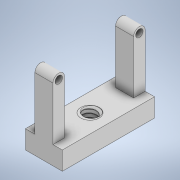
# Autodesk Inventor part: hires mount for beamsplitter test
Saved by Autodesk Inventor 2022 (Build 260153000, 153)
## iProperties
Created: 2022-07-06
Part Number: hires mount for beamsplitter test
Material: Generic
Document SubType Name: Modeling
Designer: Eli
Density: 1 g/cm^3
Appearance: Default
Author: Eli
Autodesk Inventor part; units mm, degrees
note: some values were not read from the file. Chosen so that the rebuilt part matches the saved one: direction of "Hole1"; direction of "Hole2".
ref_plane "YZ Plane" through (0, 0, 0) normal (1, 0, 0) x (0, 1, 0)
ref_plane "XZ Plane" through (0, 0, 0) normal (0, 1, 0) x (-1, 0, 0)
sketch "Sketch1" plane through (0, 0, 0) normal (0, 1, 0) x (-1, 0, 0)
  line L0 (0, 0) -> (-12.7, 0)
  line L1 (-12.7, 0) -> (-12.7, -31.75)
  line L2 (-12.7, -31.75) -> (0, -31.75)
  line L3 (0, -31.75) -> (0, 0)
  dimension "d0" = 31.75
  dimension "d1" = 12.7
  constraints: 8 end point, 2 parallel, 1 horizontal, 1 perpendicular
  measures "d0" distance of L2.end L0.start
  measures "d1" distance of L0.start L0.end
extrude "Extrusion1" add sketch "Sketch1" along normal blind 6.35
sketch "Sketch2" plane through (0, 0, 0) normal (0, -1, 0) x (1, 0, 0)
  line L0 (0, -31.75) -> (0, 0) projected
  line L1 (0, -15.875) -> (12.7, -15.875) construction
  line L2 (12.7, 0) -> (12.7, -31.75) projected
  line L3 (0, 0) -> (12.7, 0) projected
  line L4 (6.35, 0) -> (6.35, -31.75) construction
  line L5 (12.7, -31.75) -> (0, -31.75) projected
  point P0 (6.35, -15.875)
  constraints: 5 midpoint, 4 end point
hole "Hole1" at (6.35, 0, -15.875) direction (0, 1, 0) diameter 6.35 depth 6.35
thread "Thread1" size "1/4-20 UNC" class "2B" standard "ANSI Unified Screw Threads" full length
sketch "Sketch3" plane through (0, 6.35, 0) normal (0, 1, 0) x (1, 0, 0)
  line L0 (3.2385, 0) -> (9.4615, 0)
  line L1 (9.4615, 0) -> (9.4615, 3.9688)
  line L2 (9.4615, 3.9688) -> (3.2385, 3.9687)
  line L3 (3.2385, 3.9687) -> (3.2385, 0)
  line L4 (0, 0) -> (12.7, 0) construction
  line L5 (6.35, 0) -> (6.35, 31.75) construction
  line L6 (12.7, 31.75) -> (0, 31.75) construction
  line L7 (0, 31.75) -> (0, 0) construction
  line L8 (0, 15.875) -> (12.7, 15.875) construction
  line L9 (12.7, 0) -> (12.7, 31.75) construction
  line L10 (3.2385, 31.75) -> (9.4615, 31.75)
  line L11 (9.4615, 31.75) -> (9.4615, 27.7813)
  line L12 (9.4615, 27.7813) -> (3.2385, 27.7812)
  line L13 (3.2385, 27.7812) -> (3.2385, 31.75)
  dimension "d13" = 6.223
  dimension "d14" = 3.9688
  dimension "d15" = 0
  constraints: 20 end point, 4 midpoint, 4 symmetric about line, 2 parallel, 1 horizontal, 1 perpendicular, 1 other
  measures "d13" distance of L1.end L2.end
  measures "d14" distance of L0.end L1.end
  measures "d15" distance between parallel lines of L4 L0
extrude "Extrusion2" add sketch "Sketch3" along normal blind 20.32
sketch "Sketch5" plane through (9.4615, 6.35, 0) normal (1, 0, 0) x (0, 0, -1)
  line L0 (0, 0) -> (0, 20.32) construction
  line L1 (0, 18.3356) -> (3.986, 18.3356) construction
  line L2 (1.993, 18.3356) -> (1.9844, 25.4) construction
  line L3 (0, 20.32) -> (3.9688, 20.32) construction
  point P0 (0, -6.35)
  dimension "d28" = 1.9844
  constraints: 4 end point, 1 coincident, 1 horizontal, 1 midpoint, 1 point on line, 3 other
hole "Hole2" at (9.4615, 24.6856, -1.993) direction (-1, 0, 0) diameter 2.54 depth 6.223
ref_plane "Work Plane1" through (0, 6.35, -15.875) normal (0, 0, -1) x (-1, 0, 0)
mirror "Mirror1" about plane through (0, 6.35, -15.875) normal (0, 0, -1) of "Hole2"
fillet "Fillet1" radius 1.9844 4 edges at (6.35, 26.67, 0) (6.35, 26.67, -3.9688) (6.35, 26.67, -27.7813) (6.35, 26.67, -31.75)
sketch "Sketch9" plane through (6.35, 0, -15.875) normal (-1, 0, 0) x (0, 0, 1)
  line L0 (3.175, 0) -> (3.175, 6.35)
  line L1 (3.175, 6.35) -> (2.2333, 6.35)
  line L2 (2.2333, 6.35) -> (2.2333, 0)
  line L3 (2.2333, 0) -> (3.175, 0)
  line L4 (0, -7.0594) -> (0, 32.662) projected
  constraints: 8 end point
revolve "Revolution2" add sketch "Sketch9" angle 360 about axis through (6.35, 0, -15.875) along (0, 1, 0) separate body
sketch "Sketch8" plane through (6.35, 0, -12.7) normal (1, 0, 0) x (0, 1, 0)
  line L0 (-0.7409, -0.0644) -> (-0.6351, -0.0644) construction
  line L1 (0.1057, -0.8776) -> (-0.0001, -1.0809) construction
  line L2 (-1.2701, -1.0809) -> (-1.3759, -0.8776) construction
  line L3 (-0.5293, -0.0644) -> (-0.6351, 0.1389) construction
  line L4 (-0.6351, 0.1389) -> (-0.7409, -0.0644) construction
  line L5 (-1.2701, -1.0809) -> (-1.1643, -0.8776) construction
  line L6 (-0.5293, -0.0644) -> (-0.1059, -0.8776)
  line L7 (-1.3759, -0.8776) -> (-1.1643, -0.8776) construction
  arc A0 (-1.3759, -0.8776) -> (-1.2701, -0.9418) centre (-1.2701, -0.8225) ccw construction
  line L8 (0.1057, -0.8776) -> (-0.1059, -0.8776) construction
  line L9 (-1.2701, -1.0809) -> (-1.2701, -0.8776) construction
  line L10 (-0.0001, -1.0809) -> (-0.0001, -0.8776) construction
  line L11 (-0.6351, 0.1389) -> (-0.6351, -0.0002) construction
  line L12 (-1.2701, -0.9418) -> (-0.0001, -0.9418)
  arc A1 (-1.2701, -0.9418) -> (-1.1643, -0.8776) centre (-1.2701, -0.8225) ccw
  line L13 (-0.1059, -0.8776) -> (-0.0001, -1.0809) construction
  line L14 (-1.1643, -0.8776) -> (-0.7409, -0.0644)
  line L15 (-0.0001, -0.0002) -> (-0.0001, 0.0177)
  line L16 (-0.0001, 0.0177) -> (-0.0001, -0.0002)
  line L17 (-0.0001, -0.0002) -> (0.0334, -0.0002)
  arc A2 (-0.1059, -0.8776) -> (-0.0001, -0.9418) centre (-0.0001, -0.8225) ccw
  arc A3 (-0.0001, -0.9418) -> (0.1057, -0.8776) centre (-0.0001, -0.8225) ccw construction
  arc A4 (-0.6351, -0.0002) -> (-0.7409, -0.0644) centre (-0.6351, -0.1195) ccw
  arc A5 (-0.5293, -0.0644) -> (-0.6351, -0.0002) centre (-0.6351, -0.1195) ccw
  line L18 (-0.6351, -0.0002) -> (-0.6351, -0.0644) construction
  line L19 (-0.6351, -0.0644) -> (-0.5293, -0.0644) construction
  dimension "d47" = 55
  dimension "d48" = 0.2033
  dimension "d49" = 0.2033
  dimension "Sketch8_ThreadOffset" = 0
  dimension "Sketch8_MajorRadius" = 0.9417
  dimension "d52" = 1.27
  dimension "Sketch8_MinorRadius" = 0
  constraints: 40 end point, 12 point on circle, 10 parallel, 8 tangent, 6 centre point, 6 collinear, 2 midpoint, 2 point on line, 1 horizontal, 1 perpendicular, 3 other
  measures "d47" angle of L6 L14
  measures "d48" distance of L3.end L0.end
  measures "d49" distance of L1.end L10.end
  measures "Sketch8_ThreadOffset" distance between parallel lines of L15 L10
  measures "Sketch8_MajorRadius" distance from line of L12 L15.start
  measures "d52" distance from line of L1.end L9
  measures "Sketch8_MinorRadius" distance edge to line of A5 L17
coil "Coil2" sketch "Sketch8" operation cut axis through (6.35, 0, -15.875) along (0, 1, 0) pitch 1.2713 turns 6.993007 hand right bodies 2
equation "\"d47\" = d54"
equation "\"d48\" = 0.160083 * Sketch8_Pitch"
equation "\"d49\" = 0.160083 * Sketch8_Pitch"
equation "\"d52\" = Sketch8_Pitch"
equation "\"d36\" = 55deg"
equation "\"Sketch6_Pitch\" = 1.27"
equation "\"d54\" = 55deg"
equation "\"Sketch8_Pitch\" = 1.27"
body "Solid1"
body "Solid3"
